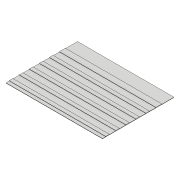
# Autodesk Inventor part: Подложка
Saved by Autodesk Inventor 2017 (Build 210142000, 142)
## iProperties
Part Number: Подложка
Material: Типовые
Document SubType Name: Modeling
Designer: Андрей
Density: 1 g/cm^3
Appearance: По умолчанию
Author: Андрей
Autodesk Inventor part; units mm, degrees
ref_plane "YZ Plane" through (0, 0, 0) normal (1, 0, 0) x (0, 1, 0)
ref_plane "XZ Plane" through (0, 0, 0) normal (0, 1, 0) x (-1, 0, 0)
ref_plane "XY Plane" through (0, 0, 0) normal (0, 0, 1) x (1, 0, 0)
sketch "Эскиз3" plane through (0, 0, 0) normal (0, 0, 1) x (1, 0, 0)
  line L0 (0, 0) -> (158.5, 0)
  line L1 (158.5, 0) -> (158.5, 117.5)
  line L2 (158.5, 117.5) -> (0, 117.5)
  line L3 (0, 117.5) -> (0, 0)
  dimension "d25" = 117.5
  dimension "d26" = 158.5
  constraints: 8 end point, 2 parallel, 1 horizontal, 1 perpendicular
  measures "d25" distance of L2.end L0.start
  measures "d26" distance of L0.start L0.end
extrude "Выдавливание2" add sketch "Эскиз3" along normal blind 1
sketch "Эскиз4" plane through (0, 0, 1) normal (0, 0, 1) x (1, 0, 0)
  line L0 (158.5, 117.5) -> (0, 117.5) projected
  line L1 (0, 117.5) -> (158.5, 117.5)
  line L2 (158.5, 117.5) -> (158.5, 97.5)
  line L3 (158.5, 97.5) -> (0, 97.5)
  line L4 (0, 97.5) -> (0, 117.5)
  line L5 (0, 117.5) -> (0, 0) projected
  line L6 (0, 87.75) -> (158.5, 87.75)
  line L7 (158.5, 87.75) -> (158.5, 77.25)
  line L8 (158.5, 77.25) -> (0, 77.25)
  line L9 (0, 77.25) -> (0, 87.75)
  line L10 (0, 71.25) -> (158.5, 71.25)
  line L11 (0, 60.75) -> (158.5, 60.75)
  line L12 (0, 54.75) -> (158.5, 54.75)
  line L13 (0, 44.25) -> (158.5, 44.25)
  line L14 (0, 38.25) -> (158.5, 38.25)
  line L15 (0, 27.75) -> (158.5, 27.75)
  line L16 (0, 21.75) -> (158.5, 21.75)
  line L17 (0, 11.25) -> (158.5, 11.25)
  line L18 (0, 5.25) -> (158.5, 5.25)
  line L19 (0, 0) -> (158.5, 0) projected
  line L20 (0, 0) -> (158.5, 0)
  line L21 (0, 71.25) -> (0, 60.75)
  line L22 (0, 54.75) -> (0, 44.25)
  line L23 (0, 38.25) -> (0, 27.75)
  line L24 (0, 21.75) -> (0, 11.25)
  line L25 (0, 5.25) -> (0, 0)
  line L26 (158.5, 0) -> (158.5, 5.25)
  line L27 (158.5, 11.25) -> (158.5, 21.75)
  line L28 (158.5, 27.75) -> (158.5, 38.25)
  line L29 (158.5, 44.25) -> (158.5, 54.75)
  line L30 (158.5, 0) -> (158.5, 117.5) projected
  line L31 (158.5, 60.75) -> (158.5, 71.25)
  dimension "d29" = 20
  dimension "d30" = 9.75
  dimension "d31" = 10.5
  dimension "d32" = 6
  dimension "d35" = 10.5
  dimension "d36" = 6
  dimension "d37" = 10.5
  dimension "d38" = 6
  dimension "d39" = 10.5
  dimension "d40" = 6
  dimension "d41" = 10.5
  dimension "d42" = 6
  dimension "d43" = 5.25
  constraints: 56 end point, 12 horizontal, 6 vertical, 4 parallel, 2 collinear, 2 perpendicular, 11 other
  measures "d29" distance between parallel lines of L3 L0
  measures "d30" distance between parallel lines of L6 L3
  measures "d31" distance between parallel lines of L8 L6
  measures "d32" distance between parallel lines of L10 L8
  measures "d35" distance between parallel lines of L11 L10
  measures "d36" distance between parallel lines of L12 L11
  measures "d37" distance between parallel lines of L13 L12
  measures "d38" distance between parallel lines of L14 L13
  measures "d39" distance between parallel lines of L15 L14
  measures "d40" distance between parallel lines of L16 L15
  measures "d41" distance between parallel lines of L17 L16
  measures "d42" distance between parallel lines of L18 L17
  measures "d43" distance between parallel lines of L19 L18
extrude "Выдавливание3" cut sketch "Эскиз4" against normal blind 0.5 contours L2 L3 L4 L0 | L7 L8 L5 L6 | L30 L11 L5 L10 | L29 L13 L5 L12 | L28 L15 L5 L14 | L27 L17 L5 L16 | L26 L19 L5 L18
